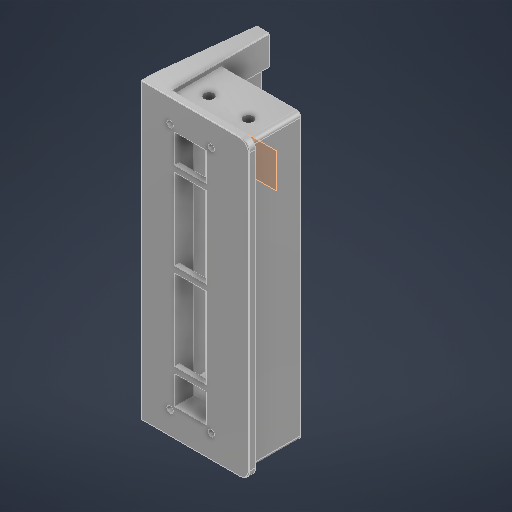
# Autodesk Inventor part: cnv_endstueck_V2
Saved by Autodesk Inventor 2026.1 (Build 301233020, 233B)
## iProperties
Created: 2025-05-08
Part Number: cnv_endstueck_V2
Material: Generisch
Document SubType Name: Modeling
Designer: iopeter
Density: 1 g/cm^3
Appearance: Gummi - Schwarz - Version 1.1
Author: iopeter
Autodesk Inventor part; units mm, degrees
ref_plane "YZ Plane" through (0, 0, 0) normal (1, 0, 0) x (0, 1, 0)
ref_plane "XZ Plane" through (0, 0, 0) normal (0, 1, 0) x (-1, 0, 0)
ref_plane "XY Plane" through (0, 0, 0) normal (0, 0, 1) x (1, 0, 0)
ref_plane "Arbeitsebene1" through (0, 0, 0) normal (0, 0, 1) x (1, 0, 0)
sketch "Skizze1" plane through (0, 0, 0) normal (0, 0, 1) x (1, 0, 0)
  line L0 (-3, -157) -> (-3, -3)
  arc A0 (-3, -3) -> (-6, 0) centre (-6, -3) ccw construction
  line L1 (-6, 0) -> (-53.3, 0) construction
  line L2 (-53.3, 0) -> (-53.3, 3) construction
  line L3 (-53.3, 3) -> (-6, 3) construction
  arc A1 (0, -3) -> (-6, 3) centre (-6, -3) ccw construction
  line L4 (0, -3) -> (0, -157)
  arc A2 (-6, -163) -> (0, -157) centre (-6, -157) ccw construction
  line L5 (-6, -163) -> (-53.3, -163) construction
  line L6 (-53.3, -163) -> (-53.3, -160) construction
  line L7 (-53.3, -160) -> (-6, -160) construction
  arc A3 (-6, -160) -> (-3, -157) centre (-6, -157) ccw construction
  line L8 (-53.3, -160) -> (-53.3, 0) construction
  line L9 (-6, -173) -> (-6, -170) projected
  line L10 (-6, -170) -> (-53.3, -170) projected
  line L11 (-53.3, -170) -> (-53.3, -173) projected
  line L12 (-53.3, -173) -> (-6, -173) projected
  line L13 (0, -167) -> (-3, -167) projected
  arc A4 (-6, -170) -> (-3, -167) centre (-6, -167) ccw projected
  line L14 (-6, -173) -> (-6, -170) projected
  arc A5 (-6, -173) -> (0, -167) centre (-6, -167) ccw projected
  line L15 (-53.3, -160) -> (-53.3, -170)
  line L16 (-3, -157) -> (-3, -167)
  line L17 (0, -157) -> (0, -167)
  line L18 (-6, 10) -> (-6, 13) projected
  line L19 (-6, 13) -> (-53.3, 13) projected
  line L20 (-53.3, 10) -> (-53.3, 13) projected
  line L21 (-53.3, 10) -> (-6, 10) projected
  line L22 (-3, 7) -> (0, 7) projected
  arc A6 (0, 7) -> (-6, 13) centre (-6, 7) ccw projected
  line L23 (-6, 10) -> (-6, 13) projected
  arc A7 (-3, 7) -> (-6, 10) centre (-6, 7) ccw projected
  line L24 (0, -167) -> (-3, -167) projected
  line L25 (0, 7) -> (0, -167) projected
  line L26 (-3, 7) -> (0, 7) projected
  line L27 (-3, 7) -> (-3, -167) projected
  line L28 (-53.3, -170) -> (-53.3, 13)
  point P0 (0, 0)
  constraints: 26 end point, 8 point on circle, 6 vertical, 4 centre point, 4 horizontal, 2 parallel, 2 tangent, 1 collinear, 20 other
extrude "Extrusion1" add sketch "Skizze1" against normal blind 32 contours L16 A4 L10 L15 L28 L21 A7 L27 L0
sketch "Skizze2" plane through (-53.3, -160, 0) normal (-1, 0, 0) x (0, 0, 1)
  line L0 (0, 163) -> (-196.7, 163) projected
  line L1 (-510, -13) -> (0, -13) projected
  line L2 (0, 170) -> (0, -10) projected
  line L3 (0, 170) -> (-32, 170) projected
  line L4 (-32, -10) -> (-32, 170) projected
  line L5 (0, -10) -> (-32, -10) projected
  line L6 (-510, 170) -> (-510, 173)
  line L7 (-510, 170) -> (0, 170)
  line L8 (0, 170) -> (0, 173)
  line L9 (0, 173) -> (-510, 173)
  line L10 (0, -13) -> (0, 173)
  line L11 (-32, -13) -> (-32, 173)
  point P0 (-32, 163)
  point P1 (0, -10)
  constraints: 12 end point, 3 point on line, 1 collinear, 1 vertical alignment
extrude "Extrusion2" add sketch "Skizze2" along normal blind 15 contours L2 L5 L4 L0 | L0 L4 L3 L2 | L3 L11 L9 L8 | L10 L1 L11 L5
ref_plane "Arbeitsebene2" through (0, 0, -2) normal (0, 0, 1) x (1, 0, 0)
ref_plane "Arbeitsebene3" through (0, 0, -2) normal (0, 0, 1) x (1, 0, 0)
sketch "Skizze7" plane through (0, 0, -32) normal (0, 0, -1) x (-1, 0, 0)
  line L0 (55.65, -49.25) -> (55.65, -110.75) projected
  line L1 (15.65, -49.25) -> (55.65, -49.25) projected
  line L2 (15.65, -110.75) -> (15.65, -49.25) projected
  line L3 (55.65, -110.75) -> (15.65, -110.75) projected
  line L4 (8, -162) -> (63.3, -162)
  line L5 (63.3, -162) -> (63.3, 2)
  line L6 (63.3, 2) -> (8, 2)
  line L7 (8, 2) -> (8, -162)
  line L8 (8, -162) -> (63.3, 2) construction
  line L9 (63.3, -162) -> (8, 2) construction
  line L10 (3, -167) -> (3, 7) projected
  line L11 (6, 10) -> (53.3, 10) projected
  line L12 (53.3, -170) -> (6, -170) projected
  point P0 (0, 0)
  point P1 (35.65, -80)
  point P2 (55.65, -80)
  point P3 (35.65, -110.75)
  point P4 (53.3, -49.25)
  point P5 (53.3, -110.75)
  dimension "d26" = 8
  constraints: 12 end point, 4 midpoint, 2 parallel, 1 horizontal, 1 horizontal alignment, 1 perpendicular, 1 vertical alignment
  measures "d26" distance between parallel lines of L11 L6
extrude "Extrusion5" cut sketch "Skizze7" against normal blind 24 contours L0 L3 L2 L1 | L7 L6 L5 L4
sketch "Skizze8" plane through (0, 0, 0) normal (0, 0, 1) x (1, 0, 0)
  line L0 (-3, -157) -> (-3, -3)
  arc A0 (-3, -3) -> (-6, 0) centre (-6, -3) ccw construction
  line L1 (-6, 0) -> (-53.3, 0) construction
  line L2 (-53.3, 0) -> (-53.3, 3) construction
  line L3 (-53.3, 3) -> (-6, 3) construction
  arc A1 (0, -3) -> (-6, 3) centre (-6, -3) ccw construction
  line L4 (0, -3) -> (0, -157)
  line L5 (-3, -167) -> (-3, -3)
  arc A2 (-3, -3) -> (-6, 0) centre (-6, -3) ccw construction
  line L6 (-6, 0) -> (-53.3, 0) construction
  line L7 (-53.3, 0) -> (-53.3, 3) construction
  line L8 (-53.3, 3) -> (-6, 3) construction
  arc A3 (0, -3) -> (-6, 3) centre (-6, -3) ccw construction
  line L9 (0, -3) -> (0, -167)
  arc A4 (-6, -173) -> (0, -167) centre (-6, -167) ccw
  line L10 (-6, -173) -> (-53.3, -173)
  line L11 (-53.3, -173) -> (-53.3, -170)
  line L12 (-53.3, -170) -> (-6, -170)
  arc A5 (-6, -170) -> (-3, -167) centre (-6, -167) ccw
  line L13 (-3, -167) -> (-3, 7) projected
  line L14 (-53.3, -170) -> (-6, -170) projected
  arc A6 (-6, -170) -> (-3, -167) centre (-6, -167) ccw projected
  arc A7 (-3, 7) -> (-6, 10) centre (-6, 7) ccw projected
  line L15 (-6, 10) -> (-53.3, 10) projected
  line L16 (-53.3, 10) -> (-53.3, 13) projected
  line L17 (-53.3, 13) -> (-68.3, 13) projected
  line L18 (-68.3, -173) -> (-68.3, 13) projected
  line L19 (-53.3, -173) -> (-68.3, -173) projected
  line L20 (-53.3, -173) -> (-53.3, -170) projected
  line L21 (0, -167) -> (-3, -167) projected
  line L22 (0, 7) -> (0, -167) projected
  line L23 (-3, 7) -> (0, 7) projected
  line L24 (-3, 7) -> (-3, -167) projected
  line L25 (-3, 7) -> (0, 7) projected
  arc A8 (0, 7) -> (-6, 13) centre (-6, 7) ccw projected
  line L26 (-6, 10) -> (-6, 13) projected
  arc A9 (-3, 7) -> (-6, 10) centre (-6, 7) ccw projected
  line L27 (-6, 10) -> (-6, 13) projected
  line L28 (-6, 13) -> (-53.3, 13) projected
  line L29 (-53.3, 10) -> (-53.3, 13) projected
  line L30 (-53.3, 10) -> (-6, 10) projected
  point P0 (0, 0)
  constraints: 26 end point, 12 point on circle, 7 vertical, 6 centre point, 6 horizontal, 21 other
extrude "Extrusion6" add sketch "Skizze8" along normal blind 4
sketch "Sketch14" plane through (0, 0, -32) normal (0, 0, -1) x (-1, 0, 0)
  line L0 (8, 2) -> (63.3, 2) projected
  line L1 (63.3, 2) -> (63.3, -162) projected
  line L2 (63.3, -162) -> (8, -162) projected
  line L3 (8, -162) -> (8, 2) projected
  line L4 (3, 7) -> (3, -167) projected
  arc A0 (3, -167) -> (6, -170) centre (6, -167) ccw projected
  line L5 (6, -170) -> (53.3, -170) projected
  line L6 (53.3, -170) -> (53.3, -173) projected
  line L7 (53.3, -173) -> (68.3, -173) projected
  line L8 (68.3, 13) -> (68.3, -173) projected
  line L9 (53.3, 13) -> (68.3, 13) projected
  line L10 (53.3, 13) -> (53.3, 10) projected
  line L11 (53.3, 10) -> (6, 10) projected
  arc A1 (6, 10) -> (3, 7) centre (6, 7) ccw projected
  line L12 (53.3, 13) -> (53.3, -173)
  line L13 (56.6, -7.5) -> (56.6, -152.5) projected
  line L14 (58.1, -6) -> (53.3, -6)
  line L15 (53.3, -6) -> (53.3, -154)
  line L16 (53.3, -154) -> (58.1, -154)
  line L17 (58.1, -154) -> (58.1, -6)
  point P0 (0, 0)
  dimension "d79" = 1.5
  dimension "d80" = 1.5
  dimension "d81" = 1.5
  constraints: 10 end point, 2 parallel, 2 perpendicular, 1 horizontal, 1 vertical alignment
  measures "d79" horizontal distance of L13.end L16.end
  measures "d80" horizontal distance of L13.end L16.end
  measures "d81" distance from line of L14 L13.start
extrude "Extrusion14" add sketch "Sketch14" along normal blind 30 contours L12 L10 L9 L8 L7 L6 L2 L1 L0 | L0 L1 L2 L12 L16 L17 L14
chamfer "Chamfer5" distance 6.7625 distance2 59.15 1 edges at (-68.3, -80, -62) measured on face at (-67.8, -80, -62)
sketch "Sketch15" plane through (-53.3, -170, -32) normal (0, -1, 0) x (1, 0, 0)
  circle A0 centre (12, 20) radius 3 construction
  circle A1 centre (37, 20) radius 3 construction
  circle A2 centre (12, 20) radius 3.2
  circle A3 centre (37, 20) radius 3.2
  point P0 (53.3, 32)
  dimension "d87" = 6.4
  dimension "d88" = 6.4
  constraints: 2 centre point, 2 coincident
  measures "d87" diameter of A2
  measures "d88" diameter of A3
extrude "Extrusion15" cut sketch "Sketch15" against normal through all
thicken "Thicken2" operation cut thickness 0.3 both sides no extend neighbours no toward (0, 1, 0) faces at (-33.1551, -170, -26.3307) (-3.4019, -168.5, -21.3333) (-3, -109, -10.6667) (-3.5213, 8.69, -21.3333) (-33.1551, 10, -26.3307)
chamfer "Chamfer6" distance 0.5 angle 45 8 edges at (-64.9187, 13, -32.425) (-53.3, 13, -31) (-68.3, 13, 0.575) (-64.9187, -173, -32.425) (-68.3, -173, 0.575) (-53.3, -173, -31) (-53.3, -154, -47) (-53.3, -6, -47)
chamfer "Chamfer7" distance 0.5 angle 45 6 edges at (-36.9, 13, 4) (-1.7574, 11.2426, 4) (0, -80, 4) (-1.7574, -171.2426, 4) (-36.9, -173, 4) (-68.3, -80, 4)
sketch "Skizze16" plane through (0, 0, 4) normal (0, 0, 1) x (1, 0, 0)
  line L0 (-67.8, -172.5) -> (-67.8, 12.5) projected
  line L1 (-6, -172.5) -> (-67.8, -172.5) projected
  arc A0 (-6, -172.5) -> (-0.5, -167) centre (-6, -167) ccw projected
  line L2 (-0.5, 7) -> (-0.5, -167) projected
  arc A1 (-0.5, 7) -> (-6, 12.5) centre (-6, 7) ccw projected
  line L3 (-67.8, 12.5) -> (-6, 12.5) projected
  line L4 (-26.9, -5) -> (-46.9, -5)
  line L5 (-46.9, -5) -> (-46.9, -155)
  line L6 (-46.9, -155) -> (-26.9, -155)
  line L7 (-26.9, -155) -> (-26.9, -5)
  line L8 (-26.9, -5) -> (-46.9, -155) construction
  line L9 (-46.9, -5) -> (-26.9, -155) construction
  point P0 (0, 0)
  point P1 (-36.9, -80)
  point P2 (-67.8, -80)
  point P3 (-36.9, 12.5)
  dimension "d99" = 20
  dimension "d100" = 150
  constraints: 12 end point, 4 midpoint, 2 parallel, 1 horizontal, 1 horizontal alignment, 1 perpendicular, 1 vertical alignment
  measures "d99" distance of L6.end L5.end
  measures "d100" distance of L5.end L4.end
extrude "Extrusion16" cut sketch "Skizze16" against normal through all contours L7 L6 L5 L4
sketch "Skizze17" plane through (0, 0, 4) normal (0, 0, 1) x (1, 0, 0)
  circle A0 centre (-49.9, -158) radius 2
  line L0 (-46.9, -5) -> (-46.9, -155) construction
  line L1 (-46.9, -80) -> (-26.9, -80) construction
  line L2 (-26.9, -155) -> (-26.9, -5) construction
  line L3 (-26.9, -155) -> (-46.9, -155) construction
  line L4 (-36.9, -155) -> (-36.9, -5) construction
  line L5 (-46.9, -5) -> (-26.9, -5) construction
  circle A1 centre (-49.9, -2) radius 2
  circle A2 centre (-23.9, -158) radius 2
  circle A3 centre (-23.9, -2) radius 2
  point P0 (0, 0)
  dimension "d103" = 4
  dimension "d104" = 3
  dimension "d105" = 3
  constraints: 4 centre point, 4 end point, 4 midpoint, 3 symmetric about line, 3 other
  measures "d103" diameter of A0
  measures "d104" horizontal distance of A0.centre L0.end
  measures "d105" horizontal distance of L0.end A0.centre
extrude "Extrusion17" cut sketch "Skizze17" against normal through all
sketch "Skizze18" plane through (0, 0, 4) normal (0, 0, 1) x (1, 0, 0)
  line L0 (-26.9, -155) -> (-26.9, -5) projected
  line L1 (-46.9, -155) -> (-46.9, -5) projected
  line L2 (-46.9, -80) -> (-26.9, -80)
  line L3 (-26.9, -78.4295) -> (-26.9, -73.4295)
  line L4 (-46.9, -69.5245) -> (-46.9, -80)
  line L5 (-46.9, -27) -> (-26.9, -27)
  line L6 (-26.9, -27) -> (-26.9, -23)
  line L7 (-26.9, -23) -> (-46.9, -23)
  line L8 (-46.9, -23) -> (-46.9, -27)
  line L9 (-46.9, -80) -> (-26.9, -80) construction
  line L10 (-46.9, -82) -> (-26.9, -82)
  line L11 (-26.9, -82) -> (-26.9, -78)
  line L12 (-26.9, -78) -> (-46.9, -78)
  line L13 (-46.9, -78) -> (-46.9, -82)
  line L14 (-26.9, -137) -> (-46.9, -137)
  line L15 (-46.9, -137) -> (-46.9, -133)
  line L16 (-46.9, -133) -> (-26.9, -133)
  line L17 (-26.9, -133) -> (-26.9, -137)
  line L18 (-26.9, -155) -> (-46.9, -155) projected
  point P0 (0, 0)
  point P1 (-26.9, -125.1896)
  point P2 (-46.9, -129.1896)
  point P3 (-46.9, -80)
  point P4 (-26.9, -23)
  point P5 (-46.9, -23)
  point P6 (-26.9, -27)
  point P7 (-26.9, -82)
  point P8 (-36.9, -155)
  point P9 (-36.9, -137)
  dimension "d111" = 4
  dimension "d112" = 4
  dimension "d116" = 4
  dimension "d117" = 18
  constraints: 32 end point, 8 point on line, 7 parallel, 5 midpoint, 5 perpendicular, 4 horizontal, 1 coincident, 1 other
  measures "d111" distance of L6.end L5.end
  measures "d112" distance of L11.end L10.end
  measures "d116" distance of L14.end L15.end
  measures "d117" distance of point (-36.9, -155) point (-36.9, -137)
extrude "Extrusion18" add sketch "Skizze18" against normal blind 3 contours L14 L1 L16 L0 | L10 L1 L2 L0 | L2 L1 L12 L0 | L5 L1 L7 L0
